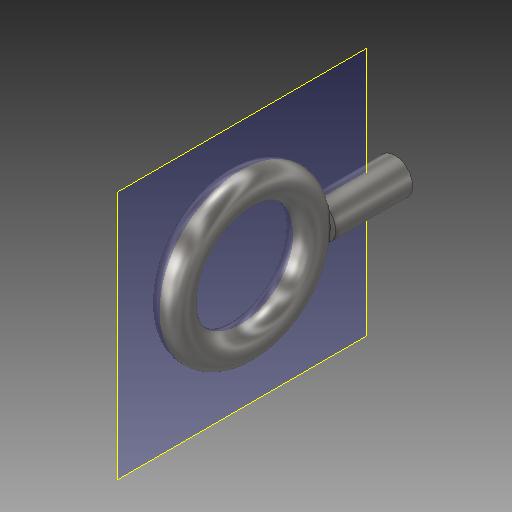
# Autodesk Inventor part: M6GBTeye
Saved by Autodesk Inventor 2019 (Build 230136000, 136)
## iProperties
Created: 2019-11-01
Part Number: M6GBTeye
Material: Stainless Steel
Document SubType Name: Modeling
Designer: Mark
Density: 8 g/cm^3
Appearance: Semi-Polished
Mass: 14.8793 g
Surface Area: 14.0977 cm^2
Volume: 1.85992 cm^3
Author: Mark
Autodesk Inventor part; units mm, degrees
ref_plane "YZ Plane" through (0, 0, 0) normal (1, 0, 0) x (0, 1, 0)
ref_plane "XZ Plane" through (0, 0, 0) normal (0, 1, 0) x (-1, 0, 0)
ref_plane "XY Plane" through (0, 0, 0) normal (0, 0, 1) x (1, 0, 0)
sketch "Sketch1" plane through (0, 0, 0) normal (0, 1, 0) x (-1, 0, 0)
  circle A0 centre (0, 11.29) radius 2.6
  line L0 (0, 11.29) -> (0, 0)
  line L1 (0, 0) -> (10, 0)
  line L2 (0, 0) -> (10, 0) construction
  dimension "d0" = 5.2
  dimension "d1" = 11.29
  dimension "d2" = 10
  constraints: 6 end point, 2 horizontal, 1 centre point, 1 collinear, 1 vertical
  measures "d0" diameter of A0
  measures "d1" distance of L0.end L0.start
  measures "d2" distance of L0.end L1.end
revolve "Revolution1" add sketch "Sketch1" angle 360 about axis through (0, 0, 0) along (-1, 0, 0)
ref_plane "Work Plane1" through (0, 0, 0) normal (-1, 0, 0) x (0, -1, 0)
sketch "Sketch2" plane through (0, 0, 0) normal (-1, 0, 0) x (0, -1, 0)
  circle A0 centre (0, 0) radius 13.89 projected
  line L0 (0, -13.89) -> (0, -25.89)
  line L1 (0, -25.89) -> (-3, -25.89)
  line L2 (-3, -25.89) -> (-3, -12.89)
  line L3 (-3, -12.89) -> (0, -12.89)
  line L4 (0, -12.89) -> (0, -25.89)
  dimension "d5" = 12
  dimension "d6" = 3
  dimension "d7" = 13
  constraints: 10 end point, 2 parallel, 1 horizontal, 1 perpendicular, 1 vertical, 1 vertical alignment, 1 other
  measures "d5" distance of L0.start L0.end
  measures "d6" distance of L2.end L3.end
  measures "d7" distance of L1.end L2.end
revolve "Revolution2" add sketch "Sketch2" angle 360 about axis through (0, 0, -13.89) along (0, 0, -1) picked at (-1.6696, -13.1747) contours L0 L1 L2 A0 | A0 L2 L3 L4
body "Solid1"
